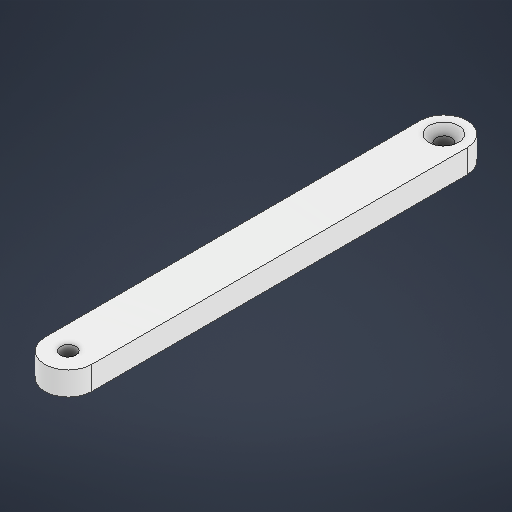
# Autodesk Inventor part: wiper_linkage_middle_arm
Saved by Autodesk Inventor 2026.2 (Build 302298000, 298)
## iProperties
Created: 2026-03-09
Part Number: wiper_linkage_middle_arm
Material: ABS Plastic
Document SubType Name: Modeling
Designer: Tathagata Sikdar
Density: 1.06 g/cm^3
Appearance: Smooth - White
Author: Tathagata Sikdar
Autodesk Inventor part; units mm, degrees
ref_plane "YZ Plane" through (0, 0, 0) normal (1, 0, 0) x (0, 1, 0)
ref_plane "XZ Plane" through (0, 0, 0) normal (0, 1, 0) x (-1, 0, 0)
ref_plane "XY Plane" through (0, 0, 0) normal (0, 0, 1) x (1, 0, 0)
sketch "Sketch1" plane through (0, 0, 0) normal (0, 1, 0) x (-1, 0, 0)
  line L0 (0, 0) -> (0, -90) construction
  line L1 (-5, -5) -> (-5, -85)
  line L2 (5, -85) -> (5, -5)
  arc A0 (5, -5) -> (-5, -5) centre (0, -5) ccw
  arc A1 (-5, -85) -> (5, -85) centre (0, -85) ccw
  circle A2 centre (0, -85) radius 1.65
  circle A3 centre (0, -5) radius 1.65
  point P0 (0, -45)
  dimension "d0" = 90
  dimension "d1" = 10
  dimension "d2" = 3.3
  constraints: 8 end point, 6 point on circle, 4 centre point, 4 tangent, 2 coincident, 2 point on line, 1 equal radius, 1 midpoint, 1 parallel, 1 vertical
  measures "d0" distance of L0.start L0.end
  measures "d1" diameter of A1
  measures "d2" diameter of A2
extrude "Extrusion1" add sketch "Sketch1" along normal blind 5
chamfer "Chamfer1" distance 1.5 angle 45 1 edges at (1.65, 5, -85)
body "Solid1"
